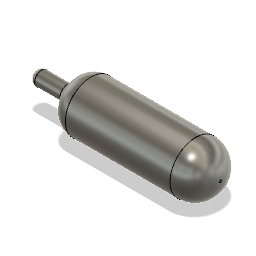
My Bottle (Autodesk Fusion 360 design; units mm, degrees)
Autodesk Fusion 360 part; units mm, degrees
sketch "Sketch1" plane through (0, 0, 0) normal (1, 0, 0) x (0, 0, -1)
  circle A0 centre (0, 0) radius 20.896
  constraint coincident A0.centre origin
extrude "Extrude1" add sketch "Sketch1" along normal blind 120
fillet "Fillet1" radius 20 1 edges at (120, -7.5563, 19.4819)
fillet "Fillet2" radius 15 1 edges at (0, -7.5563, 19.4819) 4 faces at (33.3333, -2.0806, -20.7921) (101.9011, -6.3305, -19.8189) (120, 0.3792, -0.2189) (0, 5.4457, -4.3428)
extrude "Extrude2" add 1 faces at (0, 0.2929, -0.938) along direction (-1, 0, 0) blind 30
fillet "Fillet3" radius 5 1 faces at (-20, -0.587, -5.8667)
